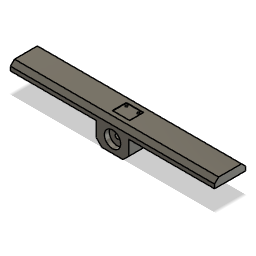
Pitch Control Lever v6 (Autodesk Fusion 360 design; units mm, degrees)
Autodesk Fusion 360 part; units mm, degrees
sketch "Sketch1" plane through (0, 0, 0) normal (0, 1, 0) x (1, 0, 0)
  line L0 (20, -19) -> (-20, -19)
  line L1 (-20, -19) -> (-20, 19)
  line L2 (-20, 19) -> (20, 19)
  line L3 (20, 19) -> (20, -19)
  line L4 (20, -19) -> (-20, 19) construction
  line L5 (-20, -19) -> (20, 19) construction
  line L6 (125, -19) -> (-125, -19)
  line L7 (-125, -19) -> (-125, 19)
  line L8 (-125, 19) -> (125, 19)
  line L9 (125, 19) -> (125, -19)
  line L10 (125, -19) -> (-125, 19) construction
  line L11 (-125, -19) -> (125, 19) construction
  dimension "d1" = 40
  dimension "d2" = 38
  dimension "d25" = 250
  dimension "d26" = 38
  constraint horizontal L0
  constraint perpendicular L0 L1
  constraint parallel L0 L2
  constraint parallel L1 L3
  constraint coincident L4 origin
  constraint coincident L5 origin
  constraint horizontal L6
  constraint perpendicular L6 L7
  constraint parallel L6 L8
  constraint parallel L7 L9
  constraint coincident L10 origin
  constraint coincident L11 origin
  measures "d1" distance of L1.end L2.end
  measures "d2" distance of L0.end L1.end
  measures "d25" distance of L7.end L8.end
  measures "d26" distance of L6.end L7.end
extrude "Extrude1" add sketch "Sketch1" along normal blind 30 contours L0 L1 L2 L3 L6 L8
sketch "Sketch3" plane through (0, 0, -19) normal (0, 0, -1) x (-1, 0, 0)
  line L0 (-20, 0) -> (20, 0)
  line L1 (20, 0) -> (20, 30)
  line L2 (-20, 30) -> (-20, 0)
  circle A0 centre (0, 20) radius 10
  circle A1 centre (0, 20) radius 2.7
  line L3 (20, 30) -> (-20, 30)
  dimension "d13" = 5.4
  constraint concentric A0 A1
  measures "d13" diameter of A1
extrude "Extrude3" cut sketch "Sketch3" against normal blind 60 contours A1
extrude "Extrude4" cut sketch "Sketch3" against normal blind 6 contours A0
extrude "Extrude5" cut sketch "Sketch3" against normal blind 6 from surface at -32 contours A0
extrude "Extrude6" add sketch "Sketch1" along normal blind 10 from surface at 30
chamfer "Chamfer2" distance 5 angle 45 4 edges at (0, 40, 19) (0, 40, -19) (0, 0, 19) (0, 0, -19)
chamfer "Chamfer3" distance 12 angle 45 2 edges at (20, 0, 0) (-20, 0, 0)
extrude "Extrude7" cut sketch "Sketch1" along normal blind 5 contours L0 L1 L2 L3 L6 L8
sketch "Sketch5" plane through (0, 40, 0) normal (0, -1, 0) x (1, 0, 0)
  line L0 (-9.9736, 7.5643) -> (-9.9736, -7.9957)
  line L1 (-9.9736, -7.9957) -> (10.2882, -7.9957)
  line L2 (10.2882, -7.9957) -> (10.2882, 7.5643)
  line L3 (10.2882, 7.5643) -> (-9.9736, 7.5643)
  circle A0 centre (-8.5238, 6.1446) radius 0.9796
  circle A1 centre (1.4942, 6.1953) radius 0.9537
  circle A2 centre (8.9673, 6.2107) radius 1.0098
  circle A3 centre (-1.0564, 6.2266) radius 0.9892
  circle A4 centre (7.6339, -5.3368) radius 1.5084
  circle A5 centre (-6.0639, 6.1567) radius 0.9903
  circle A6 centre (3.9566, 6.1712) radius 0.9784
  circle A7 centre (6.4638, 6.2006) radius 0.9737
  circle A8 centre (-3.4927, 6.169) radius 0.9564
  circle A9 centre (-7.4269, -5.3596) radius 1.4324
  line L4 (10.5, 8.5) -> (-10.5, 8.5)
  line L5 (-10.5, 8.5) -> (-10.5, -8.5)
  line L6 (-10.5, -8.5) -> (10.5, -8.5)
  line L7 (10.5, -8.5) -> (10.5, 8.5)
  line L8 (10.5, 8.5) -> (-10.5, -8.5) construction
  line L9 (-10.5, 8.5) -> (10.5, -8.5) construction
  line L10 (125, -14) -> (-125, -14)
  line L11 (-125, -14) -> (-125, 14)
  line L12 (-125, 14) -> (125, 14)
  line L13 (125, 14) -> (125, -14)
  dimension "d33" = 21
  dimension "d34" = 17
  constraint horizontal L4
  constraint perpendicular L4 L5
  constraint parallel L4 L6
  constraint parallel L5 L7
  constraint coincident L8 origin
  constraint coincident L9 origin
  measures "d33" distance of L5.end L6.end
  measures "d34" distance of L4.end L5.end
extrude "Extrude8" cut sketch "Sketch5" along normal blind 5 contours A4 | A9
extrude "Extrude9" cut sketch "Sketch5" along normal blind 0.5 contours L0 L1 L2 L3 | A0 | A1 | A2 | A3 | A5 | A6 | A7 | A8 | L4 L5 L6 L7
